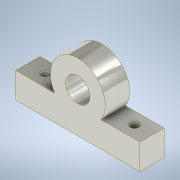
# Autodesk Inventor part: 003
Saved by Autodesk Inventor 2022.2 (Build 262287000, 287)
## iProperties
Manager: Angie Guevara
Company: ITM
Created: 2021-11-08
Part Number: 003
Material: Steel
Document SubType Name: Modeling
Designer: Samuel Gómez
Density: 7.85 g/cm^3
Appearance: Silver
Checked By: Angie Guevara
Engr Approved By: Angie Guevara
Engineer: Angie Guevara
Author: Samuel Gómez
Title: Camisa
Autodesk Inventor part; units mm, degrees
ref_plane "YZ Plane" through (0, 0, 0) normal (1, 0, 0) x (0, 1, 0)
ref_plane "XZ Plane" through (0, 0, 0) normal (0, 1, 0) x (-1, 0, 0)
ref_plane "XY Plane" through (0, 0, 0) normal (0, 0, 1) x (1, 0, 0)
sketch "Boceto1" plane through (0, 0, 0) normal (0, 0, 1) x (1, 0, 0)
  line L0 (0, 0) -> (-25.435, 0)
  line L1 (-25.435, 0) -> (-25.435, 10.53)
  line L2 (0, 0) -> (0, 11.4) construction
  arc A0 (9.5801, 10.53) -> (-9.5801, 10.53) centre (0, 16.38) ccw
  circle A1 centre (0, 16.38) radius 4.98
  line L3 (-25.435, 10.53) -> (-9.5801, 10.53)
  line L4 (0, 0) -> (25.435, 0)
  line L5 (25.435, 0) -> (25.435, 10.53)
  line L6 (25.435, 10.53) -> (9.5801, 10.53)
  dimension "d4" = 9.96
  dimension "d0" = 25.435
  dimension "d1" = 10.53
  dimension "d2" = 11.4
  dimension "d3" = 22.45
  constraints: 14 end point, 3 symmetric about line, 2 horizontal, 2 point on circle, 2 vertical, 1 centre point, 1 coincident, 1 vertical alignment, 2 other
  measures "d0" distance of L0.start L0.end
  measures "d1" distance of L0.end L1.end
  measures "d2" distance of L0.start L2.end
  measures "d3" diameter of A0
extrude "Extrusión1" add sketch "Boceto1" along normal blind 9.95
sketch "Boceto2" plane through (-25.435, 0, 0) normal (0, -1, 0) x (1, 0, 0)
  line L0 (25.435, 0) -> (25.435, 9.95) construction
  line L1 (36.66, 9.95) -> (14.21, 9.95) projected
  line L2 (25.435, 4.975) -> (41.935, 4.975) construction
  line L3 (41.935, 4.975) -> (43.685, 4.975) construction
  circle A0 centre (43.685, 4.975) radius 1.75
  circle A1 centre (7.185, 4.975) radius 1.75
  point P0 (35.0151, 9.95)
  point P1 (15.8549, 9.95)
  dimension "d7" = 16.5
  dimension "d8" = 1.75
  constraints: 6 end point, 2 horizontal, 2 midpoint, 1 centre point, 1 coincident, 1 horizontal alignment, 1 symmetric about line, 3 other
  measures "d7" distance of L2.start L2.end
  measures "d8" distance of L2.end L3.end
extrude "Extrusión2" cut sketch "Boceto2" against normal up to surface (10.53 mm away)
